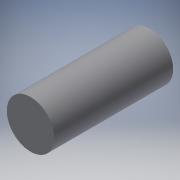
# Autodesk Inventor part: collision_cylinder_9_97
Saved by Autodesk Inventor 2018.1 (Build 221171000, 171)
## iProperties
Created: 2018-02-23
Part Number: collision_cylinder_9_97
Material: Generic
Document SubType Name: Modeling
Designer: philippe
Density: 1 g/cm^3
Appearance: Default
Author: philippe
Autodesk Inventor part; units mm, degrees
ref_plane "YZ Plane" through (0, 0, 0) normal (1, 0, 0) x (0, 1, 0)
ref_plane "XZ Plane" through (0, 0, 0) normal (0, 1, 0) x (-1, 0, 0)
ref_plane "XY Plane" through (0, 0, 0) normal (0, 0, 1) x (1, 0, 0)
sketch "Sketch1" plane through (0, 0, 0) normal (0, 1, 0) x (-1, 0, 0)
  circle A0 centre (0, 0) radius 9.97
  dimension "d0" = 19.94
  constraints: 1 centre point, 1 coincident
  measures "d0" diameter of A0
extrude "Extrusion1" add sketch "Sketch1" along normal blind 50
body "Solid1"
